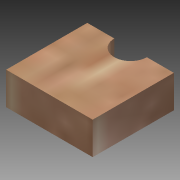
# Autodesk Inventor part: 顶杆支架
Saved by Autodesk Inventor 2013 (Build 170138000, 138)
## iProperties
Created: 2012-10-04
Part Number: 顶杆支架
Material: 木材(桦木)
Document SubType Name: Modeling
Designer: Zhensheng
Density: 7.85 g/cm^3
Author: Zhensheng
Autodesk Inventor part; units mm, degrees
ref_plane "YZ Plane" through (0, 0, 0) normal (1, 0, 0) x (0, 1, 0)
ref_plane "XZ Plane" through (0, 0, 0) normal (0, 1, 0) x (-1, 0, 0)
ref_plane "XY Plane" through (0, 0, 0) normal (0, 0, 1) x (1, 0, 0)
sketch "草图1" plane through (0, 0, 0) normal (0, 0, 1) x (1, 0, 0)
  line L0 (-4, 0) -> (4, 0)
  line L1 (-4, 0) -> (-4, 7.5)
  line L2 (4, 0) -> (4, 7.5)
  arc A0 (-1.5, 7.5) -> (1.5, 7.5) centre (0, 7.5) ccw
  line L3 (-4, 7.5) -> (-1.5, 7.5)
  line L4 (1.5, 7.5) -> (4, 7.5)
  line L5 (0, 7.5) -> (0, 0) construction
  dimension "长度" = 8
  dimension "高度" = 7.5
  dimension "d3" = 7.5
  dimension "孔径" = 3
  dimension "d5" = 7.5
  constraints: 12 end point, 2 horizontal, 2 point on circle, 2 vertical, 1 centre point, 1 coincident, 1 midpoint, 1 other
  measures "长度" distance of L0.start L0.end
  measures "高度" distance of L0.start L1.end
  measures "d3" distance of L0.end L2.end
  measures "孔径" diameter of A0
  measures "d5" distance of L5.start L5.end
extrude "拉伸1" add sketch "草图1" along normal blind 3
equation "\"d3\" = 高度"
equation "\"d5\" = 高度"
